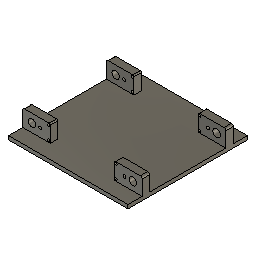
chassis (Autodesk Fusion 360 design; units mm, degrees)
Autodesk Fusion 360 part; units mm, degrees
sketch "Sketch2" plane through (0, 0, 0) normal (0, 0, 1) x (1, 0, 0)
  line L0 (-40, 40) -> (40, 40)
  line L1 (40, 40) -> (40, 0)
  line L2 (40, 0) -> (-40, 0)
  line L3 (-40, 0) -> (-40, 40)
  constraint horizontal L0
  constraint vertical L1
  constraint horizontal L2
  constraint vertical L3
extrude "Extrude2" add sketch "Sketch2" along normal blind 5 makes body 1
sketch "Sketch3" plane through (0, 0, 5) normal (0, 0, 1) x (-1, 0, 0)
  line L0 (40, 0) -> (-40, 0)
  line L1 (-40, 0) -> (-40, -40)
  line L2 (-40, -40) -> (40, -40)
  line L3 (40, -40) -> (40, 0)
  line L4 (40.4995, -21.0066) -> (3.0495, -21.0012)
  line L5 (3.0495, -21.0012) -> (3.0509, -11.0012)
  line L6 (3.0509, -11.0012) -> (40, -11.0012)
  dimension "d11" = 19
  dimension "d12" = 37.45
  dimension "d13" = 10
  constraint perpendicular L4 L5
  constraint coincident L3 L6.end
  constraint perpendicular L3 L6
  measures "d11" distance of L2.end L4.start
  measures "d12" distance of L4.start L4.end
  measures "d13" distance of L4.end L5.end
extrude "Extrude3" add sketch "Sketch3" along normal blind 22.65 contours L3 L4 L5 L6 bodies 1
sketch "Sketch4" plane through (0, 0, 0) normal (0, 1, 0) x (1, 0, 0)
  line L0 (-3.0495, -5) -> (-40, -5)
  line L1 (-40, -5) -> (-40, -27.65)
  line L2 (-40, -27.65) -> (-3.0495, -27.65)
  line L3 (-3.0495, -27.65) -> (-3.0495, -5)
  circle A0 centre (-4.9995, -25.125) radius 1.5
  circle A1 centre (-4.9995, -7.525) radius 1.5
  circle A2 centre (-16.2995, -16.325) radius 2
  circle A3 centre (-27.5495, -16.325) radius 5
  dimension "d19" = 3
  dimension "d22" = 3
  dimension "d25" = 4
  dimension "d26" = 11.25
  dimension "d27" = 10
  measures "d19" diameter of A0
  measures "d22" diameter of A1
  measures "d25" diameter of A2
  measures "d26" distance of A2.centre A3.centre
  measures "d27" diameter of A3
sketch "Sketch6" plane through (0, 0, 0) normal (0, 1, 0) x (1, 0, 0)
extrude "Extrude5" cut sketch "Sketch4" along normal blind 25 contours A0 | A1 | A2 | A3 bodies 1
fillet "Fillet3" radius 1.5 1 edges at (-3.0502, 16.0012, 27.65) on bodies 1
fillet "Fillet4" radius 2.5 1 edges at (-40, 16.0038, 27.65) on bodies 1
move_body "Move1" bodies 1 to x (1, 0, 0) y (0, 1, 0) z (0, 0, 1) at (-40, 0, 0)
move_body "Move2" bodies 1 to x (1, 0, 0) y (0, 1, 0) z (0, 0, 1) at (0, 40, 0)
mirror "Mirror1" about plane through (0, 0, 0) normal (1, 0, 0) of bodies 1 merged
mirror "Mirror2" about plane through (0, 0, 0) normal (0, 1, 0) of bodies 1 makes body 2
sketch "Sketch7" plane through (0, 0, 0) normal (0, 0, 1) x (1, 0, 0)
extrude "Extrude6" add 1 faces at (26.6667, 40, 1.6667) along direction (0, -1, 0) blind 80 on bodies 1 bodies 1 2
